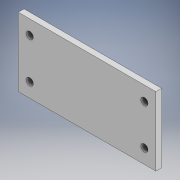
# Autodesk Inventor part: Arm Support Plate
Saved by Autodesk Inventor 2020 (Build 240168000, 168)
## iProperties
Created: 2019-10-01
Part Number: Arm Support Plate
Material: Generic
Document SubType Name: Modeling
Designer: Matt
Density: 1 g/cm^3
Appearance: Default
Author: Matt
Autodesk Inventor part; units mm, degrees
ref_plane "YZ Plane" through (0, 0, 0) normal (1, 0, 0) x (0, 1, 0)
ref_plane "XZ Plane" through (0, 0, 0) normal (0, 1, 0) x (-1, 0, 0)
ref_plane "XY Plane" through (0, 0, 0) normal (0, 0, 1) x (1, 0, 0)
sketch "Sketch1" plane through (0, 0, 0) normal (0, 0, 1) x (1, 0, 0)
  line L0 (-76.2, -38.1) -> (76.2, -38.1)
  line L1 (76.2, -38.1) -> (76.2, 38.1)
  line L2 (76.2, 38.1) -> (-76.2, 38.1)
  line L3 (-76.2, 38.1) -> (-76.2, -38.1)
  line L4 (-76.2, -38.1) -> (76.2, 38.1) construction
  line L5 (76.2, -38.1) -> (-76.2, 38.1) construction
  point P0 (0, 0)
  dimension "d0" = 152.4
  dimension "d1" = 76.2
  constraints: 12 end point, 2 midpoint, 2 parallel, 1 horizontal, 1 perpendicular
  measures "d0" distance of L2.end L1.end
  measures "d1" distance of L1.end L0.end
extrude "Extrusion1" add sketch "Sketch1" along normal blind 6.35
sketch "Sketch2" plane through (0, 0, 6.35) normal (0, 0, 1) x (1, 0, 0)
  line L0 (63.5, 0) -> (63.5, 22.225) construction
  line L1 (63.5, 22.225) -> (63.5, -22.225) construction
  line L2 (63.5, 22.225) -> (-63.5, 22.225) construction
  line L3 (-63.5, 22.225) -> (-63.5, -22.225) construction
  line L4 (-63.5, -22.225) -> (63.5, -22.225) construction
  line L5 (63.5, -22.225) -> (63.5, 22.225) construction
  point P0 (0, 0)
  dimension "d4" = 63.5
  dimension "d7" = 127
  dimension "d16" = 44.45
  dimension "d17" = 127
  dimension "d18" = 22.225
  dimension "d19" = 63.5
  constraints: 12 end point, 4 coincident, 2 parallel, 1 horizontal, 1 perpendicular, 1 point on line
  measures "d4" distance of point (0, 0) L0.start
  measures "d7" distance of L4.end L3.end
  measures "d16" distance between parallel lines of L2 L4
  measures "d17" distance of L0.end L2.end
  measures "d18" distance from line of point (0, 0) L2
  measures "d19" distance from line of point (0, 0) L3
hole "Hole1" at (-63.5, 22.225, 6.35) at (-63.5, -22.225, 6.35) at (63.5, -22.225, 6.35) at (63.5, 22.225, 6.35) direction (0, 0, -1) diameter 7.9375 depth 19.05 tip angle 118
equation "\"d18\" = 0.5 * d16"
equation "\"d19\" = 0.5 * d17"
body "Solid1"
